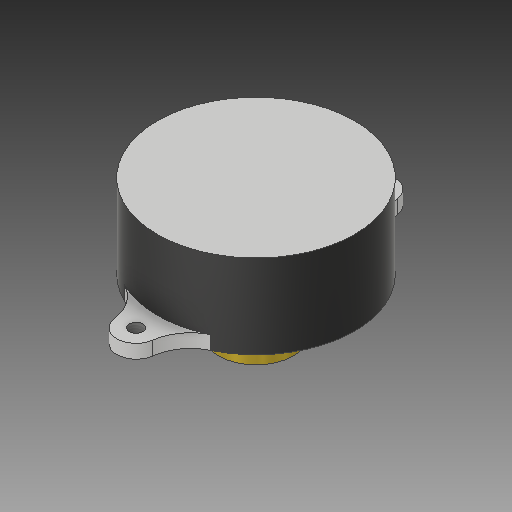
# Autodesk Inventor part: 스텝모터
Saved by Autodesk Inventor 2018 (Build 220112000, 112)
## iProperties
Created: 2018-04-03
Part Number: 스텝모터
Material: 일반
Document SubType Name: Modeling
Designer: CK
Density: 1 g/cm^3
Appearance: 기본값
Mass: 17.1522 g
Surface Area: 47.42 cm^2
Volume: 17.1522 cm^3
Author: CK
Autodesk Inventor part; units mm, degrees
ref_plane "YZ Plane" through (0, 0, 0) normal (1, 0, 0) x (0, 1, 0)
ref_plane "XZ Plane" through (0, 0, 0) normal (0, 1, 0) x (-1, 0, 0)
sketch "스케치1" plane through (0, 0, 0) normal (0, 1, 0) x (-1, 0, 0)
  circle A0 centre (0, 0) radius 18
  dimension "d0" = 36
  constraints: 1 centre point, 1 coincident
  measures "d0" diameter of A0
extrude "돌출1" add sketch "스케치1" along normal blind 12.8
sketch "스케치5" plane through (0, 0, 0) normal (0, -1, 0) x (1, 0, 0)
  arc A0 (3.4721, 22.3558) -> (-3.4721, 22.3558) centre (0, 21.915) ccw
  arc A1 (-3.4721, -22.3558) -> (3.4721, -22.3558) centre (0, -21.915) ccw
  line L0 (0, 21.915) -> (0, -21.915) construction
  circle A2 centre (0, 21.915) radius 1.25
  circle A3 centre (0, -21.915) radius 1.25
  arc A4 (3.4721, 22.3558) -> (7.8981, 16.1747) centre (11.4084, 23.3634) ccw
  arc A5 (7.8981, -16.1747) -> (3.4721, -22.3558) centre (11.4084, -23.3634) ccw
  arc A6 (-3.4721, -22.3558) -> (-7.8981, -16.1747) centre (-11.4084, -23.3634) ccw
  arc A7 (-7.8981, 16.1747) -> (-3.4721, 22.3558) centre (-11.4084, 23.3634) ccw
  circle A8 centre (0, 0) radius 18 projected
  circle A9 centre (0, 0) radius 18 projected
  dimension "d14" = 7
  dimension "d15" = 7
  dimension "d16" = 43.83
  dimension "d17" = 2.5
  dimension "d18" = 2.5
  dimension "d19" = 16
  dimension "d20" = 16
  dimension "d21" = 16
  dimension "d22" = 16
  constraints: 16 point on circle, 8 centre point, 8 tangent, 4 coincident, 2 end point, 1 midpoint, 1 vertical
  measures "d14" diameter of A0
  measures "d15" diameter of A1
  measures "d16" distance of L0.start L0.end
  measures "d17" diameter of A2
  measures "d18" diameter of A3
  measures "d19" diameter of A4
  measures "d20" diameter of A5
  measures "d21" diameter of A6
  measures "d22" diameter of A7
extrude "돌출4" add sketch "스케치5" along normal blind 2.5
thread "스레드1" size "M3x0.5" class "6H" standard "ANSI Metric M Profile" full length
thread "스레드2" size "M3x0.5" class "6H" standard "ANSI Metric M Profile" full length
sketch "스케치6" plane through (0, -2.5, 0) normal (0, -1, 0) x (1, 0, 0)
  circle A0 centre (0, 0) radius 8
  dimension "d29" = 16
  constraints: 1 centre point, 1 coincident
  measures "d29" diameter of A0
extrude "돌출5" add sketch "스케치6" along normal blind 1.85
ref_plane "작업 평면1" through (0, -6, 0) normal (0, -1, 0) x (1, 0, 0)
sketch "스케치7" plane through (0, -4.35, 0) normal (0, -1, 0) x (1, 0, 0)
  circle A0 centre (0, 0) radius 2.5
  dimension "d33" = 5
  constraints: 1 centre point, 1 coincident
  measures "d33" diameter of A0
extrude "돌출6" add sketch "스케치7" along normal blind 7.65
sketch "스케치9" plane through (0, 0, 0) normal (0, 0, 1) x (1, 0, 0)
  line L0 (-2.5, -12) -> (2.5, -12) projected
  line L1 (2.5, -12) -> (6.8309, -12)
  line L2 (6.8309, -12) -> (6.8309, -7.4987)
  line L3 (6.8309, -7.4987) -> (7.3309, -7.4987)
  line L4 (2.5, -4.35) -> (2.5, -12) projected
  line L5 (7.3309, -7.4987) -> (7.3309, -5.9987)
  line L6 (7.3309, -5.9987) -> (2.5, -5.9987)
  line L7 (0, -13.2553) -> (0, -2.7284)
  point P0 (0, 0)
  dimension "d36" = 1.5
  dimension "d37" = 0.5
  constraints: 12 end point, 3 perpendicular, 2 vertical, 1 horizontal, 1 point on line
  measures "d36" distance of L3.end L5.end
  measures "d37" distance of L2.end L3.end
revolve "회전1" add sketch "스케치9" angle 360 about axis through (0, -13.2553, 0) along (0, 1, 0)
